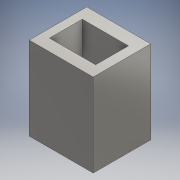
# Autodesk Inventor part: Part1
Saved by Autodesk Inventor 2016 (Build 200138000, 138)
## iProperties
Created: 2016-02-02
Part Number: Part1
Material: Steel, Alloy
Document SubType Name: Modeling
Designer: ilias
Mass: 520.341 g
Surface Area: 195.865 cm^2
Volume: 67.3144 cm^3
Density: 7.73 g/cm^3
Appearance: Semi-Polished
Author: ilias
Autodesk Inventor part; units mm, degrees
ref_plane "YZ Plane" through (0, 0, 0) normal (1, 0, 0) x (0, 1, 0)
ref_plane "XZ Plane" through (0, 0, 0) normal (0, 1, 0) x (-1, 0, 0)
ref_plane "XY Plane" through (0, 0, 0) normal (0, 0, 1) x (1, 0, 0)
sketch "Sketch1" plane through (0, 0, 0) normal (0, 0, 1) x (1, 0, 0)
  line L0 (0, 0) -> (46.0996, 0)
  line L1 (46.0996, 0) -> (46.0996, 41.4402)
  line L2 (46.0996, 41.4402) -> (0, 41.4402)
  line L3 (0, 41.4402) -> (0, 0)
  line L4 (6.0482, 32.1555) -> (39.3637, 32.1555)
  line L5 (39.3637, 32.1555) -> (39.3637, 8.4888)
  line L6 (39.3637, 8.4888) -> (6.0482, 8.4888)
  line L7 (6.0482, 8.4888) -> (6.0482, 32.1555)
  constraints: 16 end point, 4 parallel, 2 horizontal, 2 perpendicular
extrude "Extrusion1" add sketch "Sketch1" along normal blind 60
body "Solid1"
